4fee750e-2e99-4088-8574-1c80a2b96279 (Autodesk Fusion 360 design; units mm, degrees)
Autodesk Fusion 360 part; units mm, degrees
sketch "Sketch1" plane through (0, 0, 0) normal (0, 0, 1) x (1, 0, 0)
  circle A0 centre (0, 0) radius 15.875
  circle A1 centre (0, 0) radius 19.05
  dimension "d1" = 31.75
  dimension "d2" = 38.1
  measures "d1" diameter of A0
  measures "d2" diameter of A1
extrude "Extrude1" add sketch "Sketch1" along normal blind 31.75
sketch "Sketch2" plane through (0, 0, 0) normal (0, 0, -1) x (-1, 0, 0)
  circle A0 centre (0, 0) radius 19.05
  circle A1 centre (0, 0) radius 22.225
  circle A2 centre (0, 0) radius 15.875
  dimension "d5" = 44.45
  measures "d5" diameter of A1
extrude "Extrude2" add sketch "Sketch2" against normal blind 4.7625 contours A1
equation "d1 = Shaft_ID"
equation "d2 = Housing_ID"
equation "d3 = Length"
equation "d5 = Flange_OD"
equation "d6 = FlangeT"
equation "Shaft_ID = 1 1/4\""
equation "Housing_ID = 1 1/2\""
equation "FlangeT = ( -3 / 16 ) * 1 in"
equation "Length = 1 1/4\""
equation "Flange_OD = 1 3/4\""
